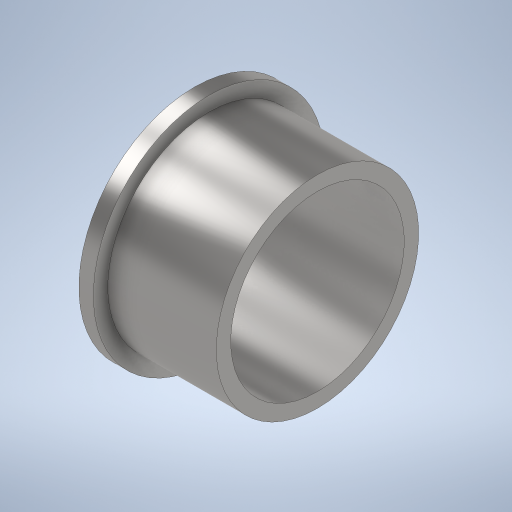
# Autodesk Inventor part: druckhusel
Saved by Autodesk Inventor 2023.2 (Build 272271000, 271)
## iProperties
Created: 2023-02-02
Part Number: druckhusel
Material: Steel, Mild
Document SubType Name: Modeling
Designer: Aditya
Density: 7.85 g/cm^3
Appearance: Semi-Polished
Author: Aditya
Autodesk Inventor part; units mm, degrees
ref_plane "YZ Plane" through (0, 0, 0) normal (1, 0, 0) x (0, 1, 0)
ref_plane "XZ Plane" through (0, 0, 0) normal (0, 1, 0) x (-1, 0, 0)
ref_plane "XY Plane" through (0, 0, 0) normal (0, 0, 1) x (1, 0, 0)
sketch "Sketch1" plane through (0, 0, 0) normal (0, 0, 1) x (1, 0, 0)
  line L0 (0, 6) -> (0, 8)
  line L1 (0, 8) -> (1, 8)
  line L2 (1, 8) -> (1, 7)
  line L3 (1, 7) -> (8.5, 7)
  line L4 (8.5, 7) -> (8.5, 6)
  line L5 (8.5, 0) -> (0, 0)
  line L6 (8.5, 7) -> (8.5, 6)
  line L7 (8.5, 6) -> (0, 6)
  dimension "d0" = 8
  dimension "d1" = 1
  dimension "d2" = 1
  dimension "d3" = 7.5
  dimension "d4" = 1
  constraints: 16 end point, 5 perpendicular, 1 horizontal, 1 vertical
  measures "d0" distance of L5.end L0.end
  measures "d1" distance of L0.end L1.end
  measures "d2" distance of L1.end L2.end
  measures "d3" distance of L2.end L3.end
  measures "d4" distance of L4.end L3.end
revolve "Revolution1" add sketch "Sketch1" angle 360 about axis through (8.5, 0, 0) along (-1, 0, 0)
body "Solid1"
